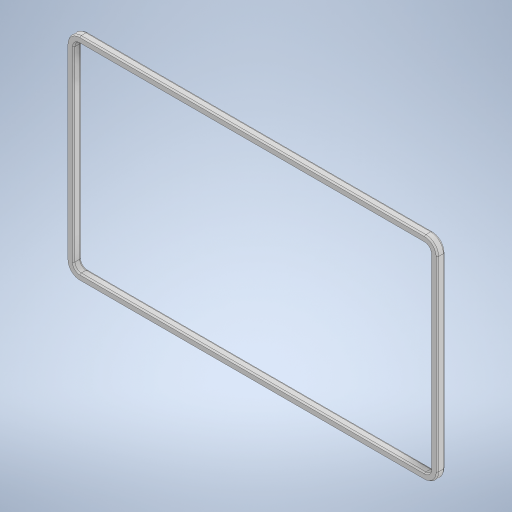
# Autodesk Inventor part: LI0012-IO SHIELD SEAL
Saved by Autodesk Inventor 2023 (Build 270158000, 158)
## iProperties
Created: 2023-04-24
Part Number: LI0012-IO SHIELD SEAL
Material: Generic
Document SubType Name: Modeling
Designer: Louis
Density: 1 g/cm^3
Appearance: Default
Author: Louis
Autodesk Inventor part; units mm, degrees
ref_plane "YZ Plane" through (0, 0, 0) normal (1, 0, 0) x (0, 1, 0)
ref_plane "XZ Plane" through (0, 0, 0) normal (0, 1, 0) x (-1, 0, 0)
ref_plane "XY Plane" through (0, 0, 0) normal (0, 0, 1) x (1, 0, 0)
sketch "Sketch1" plane through (0, 0, 0) normal (0, 0, 1) x (1, 0, 0)
  line L0 (-58.5, 33.5) -> (58.5, 33.5)
  line L1 (58.5, 33.5) -> (58.5, -33.5)
  line L2 (58.5, -33.5) -> (-58.5, -33.5)
  line L3 (-58.5, -33.5) -> (-58.5, 33.5)
  line L4 (56.5, 31.5) -> (-56.5, 31.5)
  line L5 (-56.5, 31.5) -> (-56.5, -31.5)
  line L6 (-56.5, -31.5) -> (56.5, -31.5)
  line L7 (56.5, -31.5) -> (56.5, 31.5)
  point P0 (0, 0)
  point P1 (-58.5, 0)
  point P2 (0, 33.5)
  dimension "d0" = 117
  dimension "d1" = 67
  dimension "d2" = 2
  constraints: 16 end point, 4 parallel, 2 midpoint, 2 perpendicular, 1 horizontal, 1 horizontal alignment, 1 vertical alignment, 3 other
  measures "d0" distance of L0.start L0.end
  measures "d1" distance of L0.end L1.end
  measures "d2" distance between parallel lines of L0 L4
extrude "Extrusion1" add sketch "Sketch1" along normal blind 2.5
fillet "Fillet1" radius 2 4 edges at (-56.5, 31.5, 1.25) (-56.5, -31.5, 1.25) (56.5, -31.5, 1.25) (56.5, 31.5, 1.25)
fillet "Fillet2" radius 4 4 edges at (-58.5, 33.5, 1.25) (58.5, 33.5, 1.25) (58.5, -33.5, 1.25) (-58.5, -33.5, 1.25)
chamfer "Chamfer1" distance 0.5 angle 30 8 edges at (-58.5, 0, 0) (-57.3284, -32.3284, 0) (0, -33.5, 0) (57.3284, -32.3284, 0) (58.5, 0, 0) (57.3284, 32.3284, 0) (0, 33.5, 0) (-57.3284, 32.3284, 0) measured on face at (-58.5, 0, 0.5) measured on face at (-56.9749, -31.9749, 0) measured on face at (56.9749, -31.9749, 0) measured on face at (0, 33, 0) measured on face at (-56.9749, 31.9749, 0) measured on face at (0, -33, 0) measured on face at (58, 0, 0) measured on face at (56.9749, 31.9749, 0)
chamfer "Chamfer2" distance 0.5 angle 30 8 edges at (-56.5, 0, 0) (-55.9142, 30.9142, 0) (0, 31.5, 0) (55.9142, 30.9142, 0) (56.5, 0, 0) (55.9142, -30.9142, 0) (0, -31.5, 0) (-55.9142, -30.9142, 0) measured on face at (55.9142, -30.9142, 0.5) measured on face at (-55.9142, -30.9142, 0.5) measured on face at (0, 31.5, 0.5) measured on face at (55.9142, 30.9142, 0.5) measured on face at (56.5, 0, 0.5) measured on face at (-56.5, 0, 0.5) measured on face at (0, -31.5, 0.5) measured on face at (-55.9142, 30.9142, 0.5)
chamfer "Chamfer3" distance 0.5 angle 30 8 edges at (-58.5, 0, 2.5) (-57.3284, -32.3284, 2.5) (0, -33.5, 2.5) (57.3284, -32.3284, 2.5) (58.5, 0, 2.5) (57.3284, 32.3284, 2.5) (0, 33.5, 2.5) (-57.3284, 32.3284, 2.5) measured on face at (56.9749, 31.9749, 2.5) measured on face at (-56.9749, -31.9749, 2.5) measured on face at (56.9749, -31.9749, 2.5) measured on face at (-56.9749, 31.9749, 2.5) measured on face at (-58.5, 0, 2) measured on face at (0, -33, 2.5) measured on face at (0, 33, 2.5) measured on face at (58, 0, 2.5)
chamfer "Chamfer4" distance 0.5 angle 30 8 edges at (-56.5, 0, 2.5) (-55.9142, 30.9142, 2.5) (0, 31.5, 2.5) (55.9142, 30.9142, 2.5) (56.5, 0, 2.5) (55.9142, -30.9142, 2.5) (0, -31.5, 2.5) (-55.9142, -30.9142, 2.5) measured on face at (-56.5, 0, 2) measured on face at (-55.9142, 30.9142, 2) measured on face at (0, -31.5, 2) measured on face at (55.9142, -30.9142, 2) measured on face at (0, 31.5, 2) measured on face at (55.9142, 30.9142, 2) measured on face at (-55.9142, -30.9142, 2) measured on face at (56.5, 0, 2)
body "Solid1"
